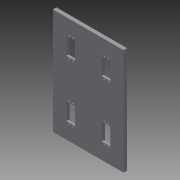
# Autodesk Inventor part: SheepBody
Saved by Autodesk Inventor 2014 SP1 (Build 180222100, 222)
## iProperties
Created: 2013-09-20
Part Number: SheepBody
Material: Generic
Document SubType Name: Modeling
Designer: Medrimonia
Density: 1 g/cm^3
Appearance: Default
ServoTraceSpacing: 0,500 mm
d73: 11,400 mm
d74: 23,500 mm
d77: 4,400 mm
d114: 11,400 mm
d115: 23,500 mm
d116: 3,000 mm
d117: 2,400 mm
d118: 4,400 mm
d121: 2,600 mm
d131: 11,400 mm
d132: 23,500 mm
d133: 4,400 mm
ServoArmWidth: 4,900 mm
ServoArmSpacing: 0,200 mm
ServoArmLength: 10,200 mm
ServoArmThickness: 1,900 mm
ServoArmHoleRequired: 3,000 mm
ServoArmHeadScrewTrace: 5,500 mm
ServoArmHeadScrewThickness: 2,500 mm
MinimalThickness: 2,000 mm
ServoArmInternFillet: 2,000 mm
ServoArmExternFillet: 2,450 mm
ServoCoreToFixation: 2,400 mm
ServoEdgeToFixation: 3,000 mm
ServoCoreWidth: 11,400 mm
ServoSpacing: 0,200 mm
ServoCoreLength: 23,500 mm
ServoFixationLength: 4,400 mm
ServoScrewDiameter: 2,000 mm
ServoScrewDiameterRequired: 2,600 mm
ServoHeadScrewTrace: 4,500 mm
ServoHeadScrewThickness: 2,500 mm
ServoExtendedSpacing: 1,000 mm
ServoAxisToCenter: 6,500 mm
BodyServoThickness: 3,000 mm
d149: 11,400 mm
d150: 23,500 mm
d151: 3,000 mm
d153: 4,400 mm
d154: 0,500 mm
d155: 0,500 mm
d158: 11,400 mm
d159: 23,500 mm
d160: 3,000 mm
d162: 4,400 mm
d183: 11,400 mm
d184: 23,500 mm
d185: 4,400 mm
d186: 0,500 mm
d187: 0,500 mm
d189: 11,400 mm
d190: 23,500 mm
d191: 4,400 mm
Author: Medrimonia
Autodesk Inventor part; units mm, degrees
ref_plane "YZ Plane" through (0, 0, 0) normal (1, 0, 0) x (0, 1, 0)
ref_plane "XZ Plane" through (0, 0, 0) normal (0, 1, 0) x (-1, 0, 0)
ref_plane "XY Plane" through (0, 0, 0) normal (0, 0, 1) x (1, 0, 0)
sketch "BodySketch" plane through (0, 0, 0) normal (0, 1, 0) x (-1, 0, 0)
  line L0 (-50, 75) -> (50, 75)
  line L1 (50, 75) -> (50, -75)
  line L2 (50, -75) -> (-50, -75)
  line L3 (-50, -75) -> (-50, 75)
  line L4 (0, 0) -> (109.854, 0) construction
  line L5 (0, 0) -> (0, -80.4744) construction
  dimension "d145" = 100
  dimension "d146" = 150
  constraints: 12 end point, 3 parallel, 2 perpendicular, 1 horizontal, 2 other
  measures "d145" distance between parallel lines of L1 L3
  measures "d146" distance between parallel lines of L2 L0
extrude "Body" add sketch "BodySketch" along normal blind 5
sketch "ServoHoles" plane through (0, 5, 0) normal (0, 1, 0) x (1, 0, 0)
  line L0 (50, -75) -> (50, 75) projected
  line L1 (19.3, 51.75) -> (30.7, 51.75) construction
  line L2 (30.7, 51.75) -> (30.7, 28.25) construction
  line L3 (30.7, 28.25) -> (19.3, 28.25) construction
  line L4 (19.3, 28.25) -> (19.3, 51.75) construction
  line L5 (19.3, 51.75) -> (19.3, 56.15) construction
  line L6 (19.3, 56.15) -> (30.7, 56.15) construction
  line L7 (30.7, 56.15) -> (30.7, 51.75) construction
  line L8 (30.7, 28.25) -> (30.7, 23.85) construction
  line L9 (30.7, 23.85) -> (19.3, 23.85) construction
  line L10 (19.3, 23.85) -> (19.3, 28.25) construction
  circle A0 centre (22.3, 54.15) radius 1.3
  line L11 (18.8, 52.25) -> (31.2, 52.25)
  line L12 (31.2, 52.25) -> (31.2, 27.75)
  line L13 (31.2, 27.75) -> (18.8, 27.75)
  line L14 (18.8, 27.75) -> (18.8, 52.25)
  line L15 (25, 69.4505) -> (25, 18.4289) construction
  line L16 (10.1912, 40) -> (43.5028, 40) construction
  circle A1 centre (27.7, 54.15) radius 1.3
  circle A2 centre (22.3, 25.85) radius 1.3
  circle A3 centre (27.7, 25.85) radius 1.3
  line L17 (0, 0) -> (0, 82.4245) construction
  line L18 (0, 0) -> (107.6133, 0) construction
  line L19 (-19.3, 51.75) -> (-30.7, 51.75) construction
  line L20 (-30.7, 51.75) -> (-30.7, 28.25) construction
  line L21 (-30.7, 28.25) -> (-19.3, 28.25) construction
  line L22 (-19.3, 28.25) -> (-19.3, 51.75) construction
  line L23 (-19.3, 51.75) -> (-19.3, 56.15) construction
  line L24 (-19.3, 56.15) -> (-30.7, 56.15) construction
  line L25 (-30.7, 56.15) -> (-30.7, 51.75) construction
  line L26 (-30.7, 28.25) -> (-30.7, 23.85) construction
  line L27 (-30.7, 23.85) -> (-19.3, 23.85) construction
  line L28 (-19.3, 23.85) -> (-19.3, 28.25) construction
  circle A4 centre (-22.3, 54.15) radius 1.3
  line L29 (-18.8, 52.25) -> (-31.2, 52.25)
  line L30 (-31.2, 52.25) -> (-31.2, 27.75)
  line L31 (-31.2, 27.75) -> (-18.8, 27.75)
  line L32 (-18.8, 27.75) -> (-18.8, 52.25)
  line L33 (-25, 69.4505) -> (-25, 18.4289) construction
  line L34 (-10.1912, 40) -> (-43.5028, 40) construction
  circle A5 centre (-27.7, 54.15) radius 1.3
  circle A6 centre (-22.3, 25.85) radius 1.3
  circle A7 centre (-27.7, 25.85) radius 1.3
  line L35 (19.3, -51.75) -> (30.7, -51.75) construction
  line L36 (30.7, -51.75) -> (30.7, -28.25) construction
  line L37 (30.7, -28.25) -> (19.3, -28.25) construction
  line L38 (19.3, -28.25) -> (19.3, -51.75) construction
  line L39 (19.3, -51.75) -> (19.3, -56.15) construction
  line L40 (19.3, -56.15) -> (30.7, -56.15) construction
  line L41 (30.7, -56.15) -> (30.7, -51.75) construction
  line L42 (30.7, -28.25) -> (30.7, -23.85) construction
  line L43 (30.7, -23.85) -> (19.3, -23.85) construction
  line L44 (19.3, -23.85) -> (19.3, -28.25) construction
  circle A8 centre (22.3, -54.15) radius 1.3
  line L45 (18.8, -52.25) -> (31.2, -52.25)
  line L46 (31.2, -52.25) -> (31.2, -27.75)
  line L47 (31.2, -27.75) -> (18.8, -27.75)
  line L48 (18.8, -27.75) -> (18.8, -52.25)
  line L49 (10.1912, -40) -> (43.5028, -40) construction
  circle A9 centre (27.7, -54.15) radius 1.3
  circle A10 centre (22.3, -25.85) radius 1.3
  circle A11 centre (27.7, -25.85) radius 1.3
  line L50 (-19.3, -51.75) -> (-30.7, -51.75) construction
  line L51 (-30.7, -56.15) -> (-30.7, -51.75) construction
  line L52 (-30.7, -51.75) -> (-30.7, -28.25) construction
  line L53 (-18.8, -52.25) -> (-31.2, -52.25)
  line L54 (-31.2, -52.25) -> (-31.2, -27.75)
  line L55 (-31.2, -27.75) -> (-18.8, -27.75)
  line L56 (-10.1912, -40) -> (-43.5028, -40) construction
  circle A12 centre (-22.3, -54.15) radius 1.3
  circle A13 centre (-27.7, -54.15) radius 1.3
  line L57 (-19.3, -28.25) -> (-19.3, -51.75) construction
  line L58 (-18.8, -27.75) -> (-18.8, -52.25)
  line L59 (-19.3, -51.75) -> (-19.3, -56.15) construction
  line L60 (-19.3, -56.15) -> (-30.7, -56.15) construction
  line L61 (-30.7, -28.25) -> (-19.3, -28.25) construction
  circle A14 centre (-27.7, -25.85) radius 1.3
  line L62 (-30.7, -28.25) -> (-30.7, -23.85) construction
  line L63 (-30.7, -23.85) -> (-19.3, -23.85) construction
  circle A15 centre (-22.3, -25.85) radius 1.3
  line L64 (-19.3, -23.85) -> (-19.3, -28.25) construction
  dimension "d149" = 11.4
  dimension "d150" = 23.5
  dimension "d151" = 3
  dimension "d153" = 4.4
  dimension "d154" = 0.5
  dimension "d155" = 0.5
  dimension "d166" = 2.4
  dimension "d167" = 2.6
  dimension "d168" = 25
  dimension "d169" = 40
  constraints: 128 end point, 59 symmetric about line, 16 centre point, 8 parallel, 7 perpendicular, 2 horizontal, 1 collinear, 20 other
  measures "d149" distance between parallel lines of L2 L4
  measures "d150" distance between parallel lines of L3 L1
  measures "d151" distance from line of L5 A0.centre
  measures "d153" distance between parallel lines of L1 L6
  measures "d154" distance between parallel lines of L1 L11
  measures "d155" distance between parallel lines of L2 L12
  measures "d166" distance from line of A0.centre L1
  measures "d167" diameter of A0
  measures "d168" distance from line of L15 L17.start
  measures "d169" distance from line of L16 L17.start
extrude "Extrusion12" cut sketch "ServoHoles" against normal through all
sketch "Sketch15" plane through (0, 5, 0) normal (0, 1, 0) x (1, 0, 0)
  line L0 (-31.2, -27.75) -> (-18.8, -27.75) projected
  line L1 (18.8, 27.75) -> (18.8, 52.25) projected
  line L2 (18.8, 52.25) -> (31.2, 52.25) projected
  line L3 (31.2, 52.25) -> (31.2, 27.75) projected
  line L4 (31.2, 27.75) -> (18.8, 27.75) projected
  circle A0 centre (-27.7, -25.85) radius 1.3 projected
  circle A1 centre (27.7, -25.85) radius 1.3 projected
  circle A2 centre (22.3, -54.15) radius 1.3 projected
  circle A3 centre (-22.3, -54.15) radius 1.3 projected
  circle A4 centre (-27.7, 25.85) radius 1.3 projected
  circle A5 centre (-22.3, 54.15) radius 1.3 projected
  circle A6 centre (22.3, 25.85) radius 1.3 projected
  circle A7 centre (22.3, 54.15) radius 1.3 projected
  circle A8 centre (27.7, 54.15) radius 1.3 projected
  circle A9 centre (27.7, 25.85) radius 1.3 projected
  circle A10 centre (-27.7, 54.15) radius 1.3 projected
  circle A11 centre (-22.3, 25.85) radius 1.3 projected
  circle A12 centre (-27.7, -54.15) radius 1.3 projected
  circle A13 centre (27.7, -54.15) radius 1.3 projected
  circle A14 centre (-22.3, -25.85) radius 1.3 projected
  circle A15 centre (22.3, -25.85) radius 1.3 projected
  line L5 (-18.8, 27.75) -> (-31.2, 27.75) projected
  line L6 (18.8, -27.75) -> (31.2, -27.75) projected
  line L7 (19.3, 51.75) -> (30.7, 51.75) construction
  line L8 (30.7, 51.75) -> (30.7, 28.25) construction
  line L9 (30.7, 28.25) -> (19.3, 28.25) construction
  line L10 (19.3, 28.25) -> (19.3, 51.75) construction
  line L11 (25, 84.5161) -> (25, -79.0915) construction
  line L12 (19.3, 51.75) -> (19.3, 56.15) construction
  line L13 (19.3, 56.15) -> (30.7, 56.15) construction
  line L14 (30.7, 56.15) -> (30.7, 51.75) construction
  line L15 (30.7, 28.25) -> (30.7, 23.85) construction
  line L16 (30.7, 23.85) -> (19.3, 23.85) construction
  line L17 (19.3, 23.85) -> (19.3, 28.25) construction
  line L18 (-1.6945, 40) -> (27.2352, 40) construction
  line L19 (18.8, 56.65) -> (31.2, 56.65)
  line L20 (31.2, 56.65) -> (31.2, 23.35)
  line L21 (31.2, 23.35) -> (18.8, 23.35)
  line L22 (18.8, 23.35) -> (18.8, 56.65)
  line L23 (25, 0) -> (25, 87.3483) construction
  line L24 (0, 0) -> (75.0033, 0) construction
  line L25 (0, 0) -> (0, 110.6198) construction
  line L26 (-18.8, 27.75) -> (-18.8, 52.25)
  line L27 (-18.8, 52.25) -> (-31.2, 52.25)
  line L28 (-31.2, 52.25) -> (-31.2, 27.75)
  line L29 (-31.2, 27.75) -> (-18.8, 27.75)
  circle A16 centre (-22.3, 25.85) radius 1.3
  circle A17 centre (-22.3, 54.15) radius 1.3
  circle A18 centre (-27.7, 54.15) radius 1.3
  circle A19 centre (-27.7, 25.85) radius 1.3
  line L30 (-19.3, 51.75) -> (-30.7, 51.75) construction
  line L31 (-30.7, 51.75) -> (-30.7, 28.25) construction
  line L32 (-30.7, 28.25) -> (-19.3, 28.25) construction
  line L33 (-19.3, 28.25) -> (-19.3, 51.75) construction
  line L34 (-19.3, 51.75) -> (-19.3, 56.15) construction
  line L35 (-19.3, 56.15) -> (-30.7, 56.15) construction
  line L36 (-30.7, 56.15) -> (-30.7, 51.75) construction
  line L37 (-30.7, 28.25) -> (-30.7, 23.85) construction
  line L38 (-30.7, 23.85) -> (-19.3, 23.85) construction
  line L39 (-19.3, 23.85) -> (-19.3, 28.25) construction
  line L40 (-18.8, 56.65) -> (-31.2, 56.65)
  line L41 (-31.2, 56.65) -> (-31.2, 23.35)
  line L42 (-31.2, 23.35) -> (-18.8, 23.35)
  line L43 (-18.8, 23.35) -> (-18.8, 56.65)
  line L44 (0, 0) -> (-75.0033, 0) construction
  line L45 (18.8, -27.75) -> (18.8, -52.25)
  line L46 (18.8, -52.25) -> (31.2, -52.25)
  line L47 (31.2, -52.25) -> (31.2, -27.75)
  line L48 (31.2, -27.75) -> (18.8, -27.75)
  circle A20 centre (-27.7, -25.85) radius 1.3
  circle A21 centre (-22.3, -54.15) radius 1.3
  circle A22 centre (22.3, -25.85) radius 1.3
  circle A23 centre (22.3, -54.15) radius 1.3
  circle A24 centre (27.7, -54.15) radius 1.3
  circle A25 centre (27.7, -25.85) radius 1.3
  circle A26 centre (-27.7, -54.15) radius 1.3
  circle A27 centre (-22.3, -25.85) radius 1.3
  line L49 (-31.2, -27.75) -> (-31.2, -52.25)
  line L50 (-31.2, -52.25) -> (-18.8, -52.25)
  line L51 (-18.8, -52.25) -> (-18.8, -27.75)
  line L52 (-18.8, -27.75) -> (-31.2, -27.75)
  line L53 (19.3, -51.75) -> (30.7, -51.75) construction
  line L54 (30.7, -51.75) -> (30.7, -28.25) construction
  line L55 (30.7, -28.25) -> (19.3, -28.25) construction
  line L56 (19.3, -28.25) -> (19.3, -51.75) construction
  line L57 (19.3, -51.75) -> (19.3, -56.15) construction
  line L58 (19.3, -56.15) -> (30.7, -56.15) construction
  line L59 (30.7, -56.15) -> (30.7, -51.75) construction
  line L60 (30.7, -28.25) -> (30.7, -23.85) construction
  line L61 (30.7, -23.85) -> (19.3, -23.85) construction
  line L62 (19.3, -23.85) -> (19.3, -28.25) construction
  line L63 (-1.6945, -40) -> (27.2352, -40) construction
  line L64 (18.8, -56.65) -> (31.2, -56.65)
  line L65 (31.2, -56.65) -> (31.2, -23.35)
  line L66 (31.2, -23.35) -> (18.8, -23.35)
  line L67 (18.8, -23.35) -> (18.8, -56.65)
  line L68 (-18.8, -27.75) -> (-18.8, -52.25)
  circle A28 centre (-22.3, -25.85) radius 1.3
  circle A29 centre (-27.7, -25.85) radius 1.3
  line L69 (-18.8, -52.25) -> (-31.2, -52.25)
  line L70 (-31.2, -52.25) -> (-31.2, -27.75)
  line L71 (-31.2, -27.75) -> (-18.8, -27.75)
  circle A30 centre (-27.7, -54.15) radius 1.3
  circle A31 centre (-22.3, -54.15) radius 1.3
  line L72 (-31.2, -23.35) -> (-18.8, -23.35)
  line L73 (-30.7, -23.85) -> (-19.3, -23.85) construction
  line L74 (-19.3, -23.85) -> (-19.3, -28.25) construction
  line L75 (-30.7, -28.25) -> (-19.3, -28.25) construction
  line L76 (-30.7, -28.25) -> (-30.7, -23.85) construction
  line L77 (-19.3, -28.25) -> (-19.3, -51.75) construction
  line L78 (-19.3, -51.75) -> (-30.7, -51.75) construction
  line L79 (-30.7, -51.75) -> (-30.7, -28.25) construction
  line L80 (-19.3, -56.15) -> (-30.7, -56.15) construction
  line L81 (-30.7, -56.15) -> (-30.7, -51.75) construction
  line L82 (-31.2, -56.65) -> (-31.2, -23.35)
  line L83 (-18.8, -56.65) -> (-31.2, -56.65)
  line L84 (-19.3, -51.75) -> (-19.3, -56.15) construction
  line L85 (-18.8, -23.35) -> (-18.8, -56.65)
  line L86 (-18.8, -27.75) -> (-18.8, -52.25) projected
  line L87 (-18.8, -52.25) -> (-31.2, -52.25) projected
  line L88 (-31.2, -52.25) -> (-31.2, -27.75) projected
  line L89 (-31.2, 27.75) -> (-31.2, 52.25) projected
  line L90 (-31.2, 52.25) -> (-18.8, 52.25) projected
  line L91 (-18.8, 52.25) -> (-18.8, 27.75) projected
  line L92 (31.2, -27.75) -> (31.2, -52.25) projected
  line L93 (31.2, -52.25) -> (18.8, -52.25) projected
  line L94 (18.8, -52.25) -> (18.8, -27.75) projected
  dimension "d183" = 11.4
  dimension "d184" = 23.5
  dimension "d185" = 4.4
  dimension "d186" = 0.5
  dimension "d187" = 0.5
  dimension "d194" = 25
  dimension "d195" = 40
  constraints: 158 end point, 55 symmetric about line, 16 centre point, 9 parallel, 7 perpendicular, 2 collinear, 2 horizontal, 1 coincident, 21 other
  measures "d183" distance between parallel lines of L8 L10
  measures "d184" distance between parallel lines of L9 L7
  measures "d185" distance between parallel lines of L7 L13
  measures "d186" distance between parallel lines of L8 L20
  measures "d187" distance between parallel lines of L13 L19
  measures "d194" distance between parallel lines of L11 L25
  measures "d195" distance between parallel lines of L24 L18
ref_plane "Work Plane9" through (0, 3, 0) normal (0, -1, 0) x (1, 0, 0)
ref_plane "Work Plane10" through (0, 5, 0) normal (0, 1, 0) x (1, 0, 0)
extrude "Extrusion14" cut sketch "Sketch15" against normal up to surface (2 mm away) from surface at 0 contours L82 L72 L85 L0 | L50 L85 L83 L82 | L4 L20 L21 L22 | L22 L19 L20 L2 | L43 L42 L41 L5 | L27 L41 L40 L43 | L67 L66 L65 L6 | L46 L65 L64 L67
equation "\"d145\" = BodyWidth"
equation "\"d146\" = BodyLength"
equation "\"d147\" = BodyThickness"
equation "\"d149\" = ServoCoreWidth"
equation "\"d150\" = ServoCoreLength"
equation "\"d151\" = ServoEdgeToFixation"
equation "\"d153\" = d162"
equation "\"d154\" = ServoTraceSpacing"
equation "\"d155\" = ServoTraceSpacing"
equation "\"d166\" = ServoCoreToFixation"
equation "\"d168\" = BodyServoWidthShift"
equation "\"d169\" = BodyServoLengthShift"
equation "\"ServoTraceSpacing\" = 0.5"
equation "\"BodyServoThickness\" = 3"
equation "\"BodyLength\" = 150"
equation "\"BodyWidth\" = 100"
equation "\"BodyThickness\" = 5"
equation "\"BodyServoWidthShift\" = 25"
equation "\"BodyServoLengthShift\" = 40"
equation "\"ServoCoreWidth\" = 11.4"
equation "\"ServoCoreLength\" = 23.5"
equation "\"ServoEdgeToFixation\" = 3"
equation "\"d162\" = 4.4"
equation "\"ServoCoreToFixation\" = 2.4"
body "Solid2"
